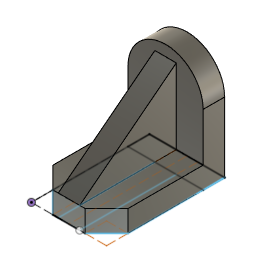
A1 piece v1 (Autodesk Fusion 360 design; units mm, degrees)
Autodesk Fusion 360 part; units mm, degrees
sketch "top view" plane through (0, 0, 0) normal (0, 0, 1) x (1, 0, 0)
  line L0 (12.0004, 0) -> (29.9996, 0)
  line L1 (42, 12) -> (42, 66)
  line L2 (42, 66) -> (0, 66)
  line L3 (0, 66) -> (0, 0) construction
  line L4 (21, 66) -> (21, 0) construction
  line L5 (0, 66) -> (15, 66)
  line L6 (15, 54) -> (15, 0)
  line L7 (15, 0) -> (12.0004, 0) construction
  line L8 (0, 12) -> (0, 66)
  line L9 (27, 54) -> (27, 0)
  line L10 (0, 0) -> (12.0004, 0) construction
  line L11 (12.0004, 0) -> (12.0004, 12) construction
  line L12 (12.0004, 12) -> (0, 12) construction
  line L13 (0, 12) -> (0, 0) construction
  line L14 (0, 12) -> (12.0004, 0)
  line L15 (29.9996, 12) -> (42, 12) construction
  line L16 (29.9996, 0) -> (29.9996, 12) construction
  line L17 (42, 12) -> (29.9996, 0)
  line L18 (42, 12) -> (42, 0) construction
  line L19 (42, 0) -> (29.9996, 0) construction
  line L20 (0, 66) -> (42, 66)
  line L21 (42, 66) -> (42, 54)
  line L22 (42, 54) -> (0, 54)
  line L23 (0, 54) -> (0, 66)
  line L24 (15, 66) -> (15, 54) construction
  line L25 (27, 54) -> (27, 66) construction
  dimension "d1" = 66
  dimension "d3" = 12
  dimension "d4" = 12
  constraint horizontal L0
  constraint vertical L1
  constraint horizontal L2
  constraint vertical L3
  constraint coincident L3.end L10.start
  constraint midpoint L2 L4.start
  constraint horizontal L5
  constraint vertical L6
  constraint horizontal L7
  constraint vertical L8
  constraint coincident L0 L6.end
  constraint symmetric L4 L6.end L9.end
  constraint horizontal L10
  constraint vertical L11
  constraint horizontal L12
  constraint vertical L13
  constraint symmetric L4 L0.start L0.end
  constraint symmetric L4 L11.end L15.start
  constraint symmetric L4 L8.start L1.start
  constraint coincident L0 L4.end
  constraint perpendicular L15 L18
  constraint perpendicular L16 L19
  constraint horizontal L20
  constraint vertical L21
  constraint horizontal L22
  constraint vertical L23
  constraint coincident L22 L6.start
  constraint coincident L22 L9.start
  constraint perpendicular L22 L24
  constraint coincident L2 L25.end
  constraint perpendicular L2 L25
  measures "d1" distance of L3.end L2.end
  measures "d3" distance of L3.end L8.start
  measures "d4" distance of L2.end L22.end
extrude "Extrude1" add sketch "top view" along normal blind 12
extrude "Extrude2" add sketch "top view" along normal blind 60 contours L1 L2 L5 L8 L20 L21 L22 L23
fillet "Fillet1" radius 21 2 edges at (0, 60, 60) (42, 60, 60)
extrude "Extrude3" add sketch "top view" along normal blind 54 contours L0 L6 L9 L22
sketch "middle part side view" plane through (0, 0, 0) normal (1, 0, 0) x (0, 1, 0)
  line L0 (0, 12) -> (54, 54)
  line L1 (54, 54) -> (54, 12)
  line L2 (54, 12) -> (0, 12)
  line L3 (0, 54) -> (0, 12)
  line L4 (54, 54) -> (0, 54)
  constraint vertical L1
  constraint perpendicular L1 L2
  constraint perpendicular L2 L3
  constraint perpendicular L3 L4
extrude "Extrude4" cut sketch "middle part side view" along normal blind 45 contours L0 L3 L4
named bodies: "A1"
